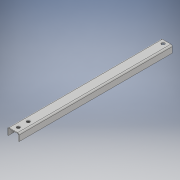
# Autodesk Inventor part: support_principal
Saved by Autodesk Inventor 2019 (Build 230136000, 136)
## iProperties
Created: 2019-03-26
Part Number: support_principal
Material: Générique
Document SubType Name: Tôle
Designer: theor
Density: 1 g/cm^3
Sheet Metal Rule: tolerie_1mm
Appearance: Par défaut
Mass: 9.79781 g
Surface Area: 202.752 cm^2
Volume: 9.79781 cm^3
Author: theor
Autodesk Inventor part; units mm, degrees
ref_plane "YZ Plane" through (0, 0, 0) normal (1, 0, 0) x (0, 1, 0)
ref_plane "XZ Plane" through (0, 0, 0) normal (0, 1, 0) x (-1, 0, 0)
ref_plane "XY Plane" through (0, 0, 0) normal (0, 0, 1) x (1, 0, 0)
sketch "Esquisse4" plane through (0, 0, 0) normal (0, 1, 0) x (-1, 0, 0)
  line L0 (-8, 108) -> (8, 108)
  line L1 (8, 108) -> (8, -108)
  line L2 (8, -108) -> (-8, -108)
  line L3 (-8, -108) -> (-8, 108)
  line L4 (-8, 108) -> (8, -108) construction
  line L5 (8, 108) -> (-8, -108) construction
  point P0 (0, 0)
  dimension "d26" = 16
  dimension "d27" = 216
  measures "d26" distance of L1.end L2.end
  measures "d27" distance of L0.end L1.end
extrude "Plaque3" add sketch "Esquisse4" along normal blind 1
sketch "Esquisse5" plane through (7, 1, 108) normal (1, 0, 0) x (0, 1, 0)
  line L0 (0, -216) -> (0, 0)
  line L1 (0, 0) -> (-10, 0)
  line L2 (-10, 0) -> (-10, -216)
  line L3 (-10, -216) -> (0, -216)
  constraints: 6 end point, 1 horizontal, 1 perpendicular, 1 vertical
edge flange "Bord tombé2" height 10 angle 90 thickness 1 bend radius 1 thickness toward (1, 0, 0) relief straight relief width 1 relief depth 0.5 corner gap 1 corner form 0 edges at (8, 0, 0) (-8, 0, 0) wall of the first edge with corners at (7, 1, -108) (7, 1, 108) (7, -9, 108) (7, -9, -108)
bend "Pli2"
corner "Coin2"
sketch "Esquisse6" plane through (0, 1, 0) normal (0, 1, 0) x (1, 0, 0)
  line L0 (-6, 108) -> (6, 108) projected
  point P0 (0, 0)
  point P1 (0, 103)
  point P2 (0, 108)
  dimension "d39" = 5
  constraints: 1 midpoint, 1 vertical alignment
  measures "d39" distance from line of L0 point (0, 103)
hole "Perçage2" at (0, 1, -103) direction (0, -1, 0) diameter 4.5 depth 1 clearance for "Vis d'assemblage à six pans creux ISO 4762" size "M4" standard "ISO"
sketch "Esquisse7" plane through (0, 1, 0) normal (0, 1, 0) x (1, 0, 0)
  line L0 (-6, 108) -> (6, 108) projected
  point P0 (0, 0)
  point P1 (0, -87)
  point P2 (0, -101)
  dimension "d50" = 195
  dimension "d51" = 14
  constraints: 2 vertical alignment
  measures "d50" distance from line of L0 point (0, -87)
  measures "d51" distance of point (0, -87) point (0, -101)
hole "Perçage3" at (0, 1, 87) at (0, 1, 101) direction (0, -1, 0) diameter 4.5 depth 1 clearance for "Vis d'assemblage à six pans creux ISO 4762" size "M4" standard "ISO"
equation "\"d45\" = Epaisseur"
equation "\"d57\" = Epaisseur"
equation "\"d28\" = Epaisseur"
equation "\"d29\" = LargeurGrugeage"
equation "\"d30\" = ProfondeurGrugeage"
equation "\"d31\" = RestesMinimum"
equation "\"d32\" = Rayondetransition"
equation "\"d35\" = RayonPli"
equation "\"d36\" = TailleGrugeage"
equation "\"d37\" = TailleJeu"
equation "\"d38\" = TailleRayonJacobi"
equation "\"RayonPli\" = Epaisseur"
equation "\"LargeurGrugeage\" = Epaisseur"
equation "\"ProfondeurGrugeage\" = 0.5 * Epaisseur"
equation "\"TailleGrugeage\" = 4 * Epaisseur"
equation "\"RestesMinimum\" = 2 * Epaisseur"
equation "\"Rayondetransition\" = RayonPli"
equation "\"TailleRayonJacobi\" = RayonPli"
equation "\"TailleJeu\" = Epaisseur"
equation "\"Epaisseur\" = 1"
